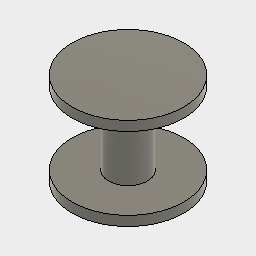
Top&WheelConnector (Autodesk Fusion 360 design; units mm, degrees)
Autodesk Fusion 360 part; units mm, degrees
sketch "Sketch5" plane through (0, 0, 0) normal (0, 1, 0) x (1, 0, 0)
  circle A0 centre (0, 0) radius 11.5
  circle A1 centre (0, 0) radius 4
  dimension "d23" = 23
  dimension "d24" = 8
  constraint coincident A0.centre A1.centre
  constraint concentric A0 A1
  measures "d23" diameter of A0
  measures "d24" diameter of A1
extrude "Extrude7" add sketch "Sketch5" along normal blind 25 contours A1 makes body 1
extrude "Extrude8" add sketch "Sketch5" along normal blind 5 bodies 1
sketch "Sketch6" plane through (0, 25, 0) normal (0, 1, 0) x (-1, 0, 0)
  circle A0 centre (0, 0) radius 4
  circle A1 centre (0, 0) radius 11.5
  dimension "d29" = 23
  constraint coincident A0.centre A1.centre
  measures "d29" diameter of A1
extrude "Extrude9" add sketch "Sketch6" against normal blind 5 bodies 1
extrude "Extrude10" cut 1 faces at (8.9423, 5, 0.7701) along direction (0, -1, 0) blind 3 on bodies 1 bodies 1
extrude "Extrude11" add 1 faces at (-0.7598, 25, -3.4999) along direction (0, -1, 0) blind 7 separate body on bodies 1 makes body 2
extrude "Extrude12" cut 1 faces at (-0.7598, 25, -3.4999) along direction (0, -1, 0) blind 5 on bodies 1 bodies 1 2
extrude "Extrude13" add 1 faces at (-0.7598, 20, -3.4999) along direction (0, 1, 0) blind 1 on bodies 2 bodies 2 1
extrude "Extrude14" add 1 faces at (-0.7598, 21, -3.4999) along direction (0, 1, 0) blind 1 on bodies 2 bodies 2
extrude "Extrude15" cut 1 faces at (-0.7598, 22, -3.4999) along direction (0, -1, 0) blind 2 on bodies 2 bodies 2
extrude "Extrude16" add 1 faces at (-8.9423, 18, -0.7701) along direction (0, -1, 0) blind 1 on bodies 2 bodies 2
extrude "Extrude17" cut 1 faces at (-0.7598, 20, -3.4999) along direction (0, -1, 0) blind 1 on bodies 2 bodies 2
copy_body "Body->Comp2" bodies 2 removing the originals makes body 3 in component "Axle Connector"
component "Axle Connector" placed x (1, 0, 0) y (0, 1, 0) z (0, 0, 1) at (0, 0, 0)
named bodies: "Axle Connector"
